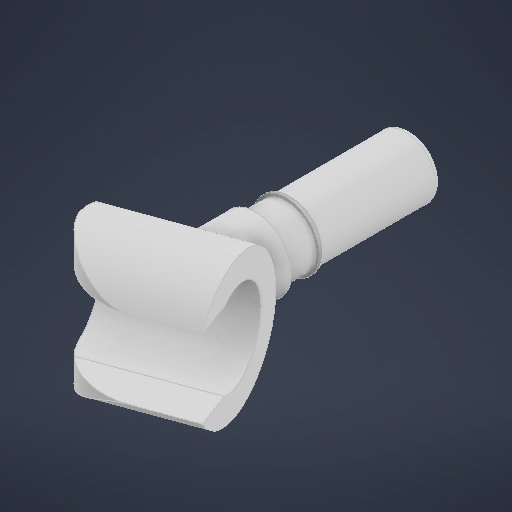
# Autodesk Inventor part: Lego hand
Saved by Autodesk Inventor 2027.1 (Build 311270010, 270A)
## iProperties
Created: 2020-11-13
Part Number: Lego hand
Material: Generic
Document SubType Name: Modeling
Designer: 164344
Density: 1 g/cm^3
Appearance: Default
Author: 164344
Autodesk Inventor part; units mm, degrees
sketch "Sketch1" plane through (0, 0, 0) normal (0, 0, 1) x (1, 0, 0)
  circle A0 centre (0, 0) radius 1.1
  dimension "d0" = 2.2
  constraints: 1 centre point, 1 coincident
  measures "d0" diameter of A0
extrude "Extrusion1" add sketch "Sketch1" along normal blind 5.6
ref_plane "Work Plane1" through (0, 0, 4.5) normal (0, 0, 1) x (1, 0, 0)
sketch "Sketch2" plane through (0, 0, 4.5) normal (0, 0, 1) x (1, 0, 0)
  circle A0 centre (0, 0) radius 1.1 projected
  circle A1 centre (0, 0) radius 1.2
  dimension "d4" = 0.1
  constraints: 1 centre point
  measures "d4" radial gap between concentric circles of A0 A1
extrude "Extrusion2" add sketch "Sketch2" against normal blind 0.2
chamfer "Chamfer1" distance 0.1 angle 45 1 edges at (-1.2, 0, 4.3)
fillet "Fillet1" radius 0.2 1 edges at (-1.1, 0, 0)
sketch "Sketch3" plane through (0, 0, 5.6) normal (0, 0, 1) x (1, 0, 0)
  circle A0 centre (0, 0) radius 1.1 projected
  circle A1 centre (0, 0) radius 1.3
  dimension "d11" = 0.2
  constraints: 1 centre point
  measures "d11" radial gap between concentric circles of A0 A1
extrude "Extrusion3" add sketch "Sketch3" along normal blind 3 contours A0 | A1
ref_plane "Work Plane3" through (-4.9804, 0, 1.8127) normal (0.9396926, 0, -0.3420201) x (0, 1, 0)
ref_plane "Work Plane2" through (0, 0, 0) normal (0.9396926, 0, -0.3420201) x (0, 1, 0)
sketch "Sketch4" plane through (-4.9804, 0, 1.8127) normal (0.9396926, 0, -0.3420201) x (0, 1, 0)
  ellipse E0 centre (0, 5.2623) end of major axis (1.3, 5.2623) minor radius 0.4446 projected
  line L0 (-1.3, 5.2623) -> (-1.3, 8.0814) projected
  circle A0 centre (0, 8.8623) radius 2.45
  point P0 (0, 0)
  dimension "d16" = 4.9
  dimension "d17" = 3.6
  dimension "d18" = 1.3
  constraints: 1 centre point, 1 horizontal alignment
  measures "d16" diameter of A0
  measures "d17" distance of A0.centre point (0, 5.262)
  measures "d18" distance from line of L0 A0.centre
extrude "Extrusion4" add sketch "Sketch4" along normal blind 4.5 contours A0
sketch "Sketch5" plane through (-1.9493, 0, 10.1405) normal (-0.9396926, 0, 0.3420201) x (0.3420201, 0, 0.9396926)
  circle A0 centre (0, 0) radius 2.45 projected
  arc A1 (0.6652, 1.4) -> (0.6652, -1.4) centre (0, 0) ccw
  line L0 (0.6652, 1.4) -> (3.89, 1.4)
  line L1 (3.89, 1.4) -> (3.89, -1.4)
  line L2 (3.89, -1.4) -> (0.6652, -1.4)
  point P0 (-8.8623, 0)
  dimension "d21" = 0.9
  dimension "d22" = 1.4
  dimension "d23" = 1.4
  dimension "d25" = 3.89
  constraints: 6 end point, 2 perpendicular, 2 point on circle, 1 centre point, 1 horizontal
  measures "d21" radial gap between concentric circles of A0 A1
  measures "d22" distance from line of L2 A0.centre
  measures "d23" distance from line of L0 A0.centre
  measures "d25" distance from line of L1 A0.centre
extrude "Extrusion5" cut sketch "Sketch5" against normal blind 4.5 contours A0 L2 A1 L0 | A0 L0 L1 L2 picked at (1.2601, 0)
ref_plane "Work Plane4" through (0, 3, 0) normal (0, 1, 0) x (-1, 0, 0)
sketch "Sketch6" plane through (0, 3, 0) normal (0, 1, 0) x (-1, 0, 0)
  line L0 (-1.0876, 11.1748) -> (1.2616, 12.0299)
  line L1 (2.0243, 9.9344) -> (1.2616, 12.0299)
  arc A0 (2.0243, 9.9344) -> (-1.0876, 11.1748) centre (-0.227, 8.8102) ccw
  point P0 (0, 0)
  dimension "d29" = 2.5
  dimension "d30" = 2.23
  constraints: 4 end point, 2 point on circle, 1 centre point, 1 tangent
  measures "d29" distance from line of L1 L0.start
  measures "d30" distance from line of L0 L1.start
extrude "Extrusion6" cut sketch "Sketch6" against normal through all
body "Solid1"
